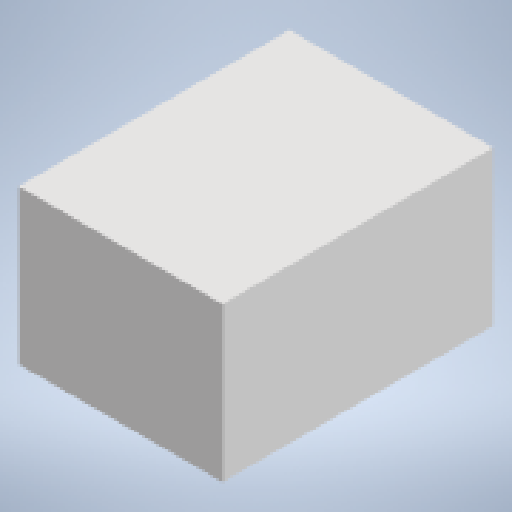
# Autodesk Inventor part: деталь будет крепить ремень
Saved by Autodesk Inventor 2024.2 (Build 282272000, 272)
## iProperties
Created: 2026-02-03
Part Number: деталь будет крепить ремень
Material: Типовые
Document SubType Name: Modeling
Designer: katya_notebook
Density: 1 g/cm^3
Appearance: По умолчанию
Author: katya_notebook
Autodesk Inventor part; units mm, degrees
ref_plane "YZ Plane" through (0, 0, 0) normal (1, 0, 0) x (0, 1, 0)
ref_plane "XZ Plane" through (0, 0, 0) normal (0, 1, 0) x (-1, 0, 0)
ref_plane "XY Plane" through (0, 0, 0) normal (0, 0, 1) x (1, 0, 0)
sketch "Эскиз1" plane through (0, 0, 0) normal (0, 0, 1) x (1, 0, 0)
  line L0 (4.9701, 7.2976) -> (4.9701, 8.7976)
  line L1 (4.9701, 8.7976) -> (-3.0052, 8.7976)
  line L2 (-3.0052, 7.2976) -> (4.9701, 7.2976)
  line L3 (-3.0052, 8.7976) -> (-3.0052, 7.2976)
  line L4 (-3.0052, 5.7776) -> (4.9701, 5.7776)
  line L5 (4.9701, 5.7776) -> (4.9701, 4.2776)
  line L6 (4.9701, 4.2776) -> (-3.0052, 4.2776)
  line L7 (-3.0052, 4.2776) -> (-3.0052, 5.7776)
  line L8 (4.9701, 5.0276) -> (-5.8657, 5.0276)
  arc A0 (-3.0052, 2.7576) -> (-2.4573, 3.2802) centre (-3.0114, 3.3126) ccw
  line L9 (-3.0052, 2.7576) -> (-3.0104, 4.0302)
  line L10 (-3.0104, 4.0302) -> (-3.0104, 4.2776)
  line L11 (-1.0104, 4.2776) -> (-1.0104, 3.8676)
  arc A1 (-1.0104, 3.8676) -> (-1.0114, 3.8676) centre (-1.0114, 3.3126) ccw
  line L12 (-1.0114, 3.8676) -> (-1.0114, 2.7576)
  arc A2 (-1.5664, 3.311) -> (-1.0114, 2.7576) centre (-1.0114, 3.3126) ccw
  line L13 (-1.5664, 3.311) -> (-1.5664, 3.3135)
  arc A3 (-1.5647, 3.3559) -> (-1.5664, 3.3135) centre (-1.0114, 3.3126) ccw
  arc A4 (-1.5647, 3.3559) -> (-1.7142, 3.5176) centre (-1.7142, 3.3676) ccw
  line L14 (-1.7142, 3.5176) -> (-2.3054, 3.5176)
  arc A5 (-2.3054, 3.5176) -> (-2.4554, 3.3676) centre (-2.3054, 3.3676) ccw
  line L15 (-2.4554, 3.3676) -> (-2.4554, 3.2802)
  line L16 (-2.4554, 3.2802) -> (-2.4573, 3.2802)
  arc A6 (-1.0114, 2.7576) -> (-0.4635, 3.2802) centre (-1.0175, 3.3126) ccw
  line L17 (-1.0114, 2.7576) -> (-1.0166, 4.0302)
  line L18 (-1.0166, 4.0302) -> (-1.0166, 4.2776)
  line L19 (0.9834, 4.2776) -> (0.9834, 3.8676)
  arc A7 (0.9834, 3.8676) -> (0.9825, 3.8676) centre (0.9825, 3.3126) ccw
  line L20 (0.9825, 3.8676) -> (0.9825, 2.7576)
  arc A8 (0.4275, 3.311) -> (0.9825, 2.7576) centre (0.9825, 3.3126) ccw
  line L21 (0.4275, 3.311) -> (0.4275, 3.3135)
  arc A9 (0.4291, 3.3559) -> (0.4275, 3.3135) centre (0.9825, 3.3126) ccw
  arc A10 (0.4291, 3.3559) -> (0.2796, 3.5176) centre (0.2796, 3.3676) ccw
  line L22 (0.2796, 3.5176) -> (-0.3116, 3.5176)
  arc A11 (-0.3116, 3.5176) -> (-0.4616, 3.3676) centre (-0.3116, 3.3676) ccw
  line L23 (-0.4616, 3.3676) -> (-0.4616, 3.2802)
  line L24 (-0.4616, 3.2802) -> (-0.4635, 3.2802)
  arc A12 (0.9825, 2.7576) -> (1.5304, 3.2802) centre (0.9763, 3.3126) ccw
  line L25 (0.9825, 2.7576) -> (0.9772, 4.0302)
  line L26 (0.9772, 4.0302) -> (0.9772, 4.2776)
  line L27 (2.9772, 4.2776) -> (2.9772, 3.8676)
  arc A13 (2.9772, 3.8676) -> (2.9763, 3.8676) centre (2.9763, 3.3126) ccw
  line L28 (2.9763, 3.8676) -> (2.9763, 2.7576)
  arc A14 (2.4213, 3.311) -> (2.9763, 2.7576) centre (2.9763, 3.3126) ccw
  line L29 (2.4213, 3.311) -> (2.4213, 3.3135)
  arc A15 (2.423, 3.3559) -> (2.4213, 3.3135) centre (2.9763, 3.3126) ccw
  arc A16 (2.423, 3.3559) -> (2.2734, 3.5176) centre (2.2734, 3.3676) ccw
  line L30 (2.2734, 3.5176) -> (1.6822, 3.5176)
  arc A17 (1.6822, 3.5176) -> (1.5322, 3.3676) centre (1.6822, 3.3676) ccw
  line L31 (1.5322, 3.3676) -> (1.5322, 3.2802)
  line L32 (1.5322, 3.2802) -> (1.5304, 3.2802)
  arc A18 (2.9763, 2.7576) -> (3.5242, 3.2802) centre (2.9701, 3.3126) ccw
  line L33 (2.9763, 2.7576) -> (2.9711, 4.0302)
  line L34 (2.9711, 4.0302) -> (2.9711, 4.2776)
  line L35 (4.9711, 4.2776) -> (4.9711, 3.8676)
  arc A19 (4.9711, 3.8676) -> (4.9701, 3.8676) centre (4.9701, 3.3126) ccw
  line L36 (4.9701, 3.8676) -> (4.9701, 2.7576)
  arc A20 (4.4151, 3.311) -> (4.9701, 2.7576) centre (4.9701, 3.3126) ccw
  line L37 (4.4151, 3.311) -> (4.4151, 3.3135)
  arc A21 (4.4168, 3.3559) -> (4.4151, 3.3135) centre (4.9701, 3.3126) ccw
  arc A22 (4.4168, 3.3559) -> (4.2673, 3.5176) centre (4.2673, 3.3676) ccw
  line L38 (4.2673, 3.5176) -> (3.6761, 3.5176)
  arc A23 (3.6761, 3.5176) -> (3.5261, 3.3676) centre (3.6761, 3.3676) ccw
  line L39 (3.5261, 3.3676) -> (3.5261, 3.2802)
  line L40 (3.5261, 3.2802) -> (3.5242, 3.2802)
  line L41 (4.9701, 2.7576) -> (-3.0052, 2.7576)
  line L42 (-3.0052, 2.7576) -> (-3.0052, 1.2576)
  line L43 (-3.0052, 1.2576) -> (4.9701, 1.2576)
  line L44 (4.9701, 1.2576) -> (4.9701, 2.7576)
  line L45 (-2.3054, 3.5176) -> (5.394, 3.5176)
  line L46 (4.9701, 3.7226) -> (4.3774, 3.7226)
  arc A24 (-0.4635, 3.755) -> (-1.0114, 4.2776) centre (-1.0175, 3.7226) ccw
  line L47 (0.9825, 4.2776) -> (0.9772, 3.005)
  line L48 (0.9825, 3.1676) -> (0.9825, 4.2776)
  line L49 (-1.0114, 4.2776) -> (-1.0166, 3.005)
  arc A25 (-2.4573, 3.755) -> (-3.0052, 4.2776) centre (-3.0114, 3.7226) ccw
  line L50 (-1.0114, 3.1676) -> (-1.0114, 4.2776)
  arc A26 (-1.5664, 3.7217) -> (-1.5647, 3.6793) centre (-1.0114, 3.7226) ccw
  line L51 (-1.5664, 3.7241) -> (-1.5664, 3.7217)
  arc A27 (-1.0114, 4.2776) -> (-1.5664, 3.7241) centre (-1.0114, 3.7226) ccw
  arc A28 (-1.7142, 3.5176) -> (-1.5647, 3.6793) centre (-1.7142, 3.6676) ccw
  arc A29 (1.5304, 3.755) -> (0.9825, 4.2776) centre (0.9763, 3.7226) ccw
  arc A30 (2.4213, 3.7217) -> (2.423, 3.6793) centre (2.9763, 3.7226) ccw
  arc A31 (2.9763, 4.2776) -> (2.4213, 3.7241) centre (2.9763, 3.7226) ccw
  line L52 (2.9763, 4.2776) -> (2.9711, 3.005)
  arc A32 (-2.4554, 3.6676) -> (-2.3054, 3.5176) centre (-2.3054, 3.6676) ccw
  line L53 (-2.4554, 3.6676) -> (-2.4554, 3.755)
  line L54 (-2.4554, 3.755) -> (-2.4573, 3.755)
  arc A33 (0.9825, 4.2776) -> (0.4275, 3.7241) centre (0.9825, 3.7226) ccw
  line L55 (0.4275, 3.7241) -> (0.4275, 3.7217)
  arc A34 (0.4275, 3.7217) -> (0.4291, 3.6793) centre (0.9825, 3.7226) ccw
  arc A35 (-0.4616, 3.6676) -> (-0.3116, 3.5176) centre (-0.3116, 3.6676) ccw
  line L56 (-0.4616, 3.755) -> (-0.4635, 3.755)
  arc A36 (0.2796, 3.5176) -> (0.4291, 3.6793) centre (0.2796, 3.6676) ccw
  line L57 (2.9763, 3.1676) -> (2.9763, 4.2776)
  line L58 (3.5261, 3.755) -> (3.5242, 3.755)
  line L59 (3.5261, 3.6676) -> (3.5261, 3.755)
  arc A37 (3.5261, 3.6676) -> (3.6761, 3.5176) centre (3.6761, 3.6676) ccw
  arc A38 (3.5242, 3.755) -> (2.9763, 4.2776) centre (2.9701, 3.7226) ccw
  arc A39 (4.9701, 4.2776) -> (4.4151, 3.7241) centre (4.9701, 3.7226) ccw
  line L60 (-0.4616, 3.6676) -> (-0.4616, 3.755)
  arc A40 (2.2734, 3.5176) -> (2.423, 3.6793) centre (2.2734, 3.6676) ccw
  line L61 (2.4213, 3.7241) -> (2.4213, 3.7217)
  line L62 (4.4151, 3.7241) -> (4.4151, 3.7217)
  arc A41 (4.4151, 3.7217) -> (4.4168, 3.6793) centre (4.9701, 3.7226) ccw
  arc A42 (1.5322, 3.6676) -> (1.6822, 3.5176) centre (1.6822, 3.6676) ccw
  line L63 (1.5322, 3.755) -> (1.5304, 3.755)
  arc A43 (4.2673, 3.5176) -> (4.4168, 3.6793) centre (4.2673, 3.6676) ccw
  line L64 (1.5322, 3.6676) -> (1.5322, 3.755)
  line L65 (4.9701, 3.3126) -> (4.3774, 3.3126)
  line L66 (4.9701, 4.2776) -> (4.9701, 5.7776)
  line L67 (4.9701, 5.7776) -> (-3.0052, 5.7776)
  line L68 (-3.0052, 5.7776) -> (-3.0052, 4.2776)
  arc A44 (-1.0114, 6.1876) -> (-1.0104, 6.1876) centre (-1.0114, 6.7426) ccw
  arc A45 (-0.4635, 6.775) -> (-1.0114, 7.2976) centre (-1.0175, 6.7426) ccw
  line L69 (0.9825, 7.2976) -> (0.9772, 6.025)
  line L70 (0.9825, 6.1876) -> (0.9825, 7.2976)
  line L71 (0.9772, 6.025) -> (0.9772, 5.7776)
  line L72 (-1.0104, 5.7776) -> (-1.0104, 6.1876)
  line L73 (-1.0114, 7.2976) -> (-1.0166, 6.025)
  line L74 (-1.0166, 6.025) -> (-1.0166, 5.7776)
  line L75 (-3.0104, 6.025) -> (-3.0104, 5.7776)
  line L76 (-3.0052, 7.2976) -> (-3.0104, 6.025)
  arc A46 (-2.4573, 6.775) -> (-3.0052, 7.2976) centre (-3.0114, 6.7426) ccw
  line L77 (-1.0114, 6.1876) -> (-1.0114, 7.2976)
  arc A47 (-1.5664, 6.7417) -> (-1.5647, 6.6993) centre (-1.0114, 6.7426) ccw
  line L78 (-1.5664, 6.7441) -> (-1.5664, 6.7417)
  arc A48 (-1.0114, 7.2976) -> (-1.5664, 6.7441) centre (-1.0114, 6.7426) ccw
  arc A49 (-1.7142, 6.5376) -> (-1.5647, 6.6993) centre (-1.7142, 6.6876) ccw
  line L79 (0.9834, 5.7776) -> (0.9834, 6.1876)
  arc A50 (0.9825, 6.1876) -> (0.9834, 6.1876) centre (0.9825, 6.7426) ccw
  arc A51 (1.5304, 6.775) -> (0.9825, 7.2976) centre (0.9763, 6.7426) ccw
  arc A52 (2.4213, 6.7417) -> (2.423, 6.6993) centre (2.9763, 6.7426) ccw
  arc A53 (2.9763, 7.2976) -> (2.4213, 6.7441) centre (2.9763, 6.7426) ccw
  line L80 (2.9763, 7.2976) -> (2.9711, 6.025)
  line L81 (2.9772, 5.7776) -> (2.9772, 6.1876)
  line L82 (2.9711, 6.025) -> (2.9711, 5.7776)
  line L83 (-1.7142, 6.5376) -> (-2.3054, 6.5376)
  arc A54 (-2.4554, 6.6876) -> (-2.3054, 6.5376) centre (-2.3054, 6.6876) ccw
  line L84 (-2.4554, 6.6876) -> (-2.4554, 6.775)
  line L85 (-2.4554, 6.775) -> (-2.4573, 6.775)
  arc A55 (0.9825, 7.2976) -> (0.4275, 6.7441) centre (0.9825, 6.7426) ccw
  line L86 (0.4275, 6.7441) -> (0.4275, 6.7417)
  arc A56 (0.4275, 6.7417) -> (0.4291, 6.6993) centre (0.9825, 6.7426) ccw
  line L87 (0.2796, 6.5376) -> (-0.3116, 6.5376)
  arc A57 (-0.4616, 6.6876) -> (-0.3116, 6.5376) centre (-0.3116, 6.6876) ccw
  line L88 (-0.4616, 6.775) -> (-0.4635, 6.775)
  arc A58 (0.2796, 6.5376) -> (0.4291, 6.6993) centre (0.2796, 6.6876) ccw
  line L89 (2.9763, 6.1876) -> (2.9763, 7.2976)
  line L90 (3.5261, 6.775) -> (3.5242, 6.775)
  line L91 (3.5261, 6.6876) -> (3.5261, 6.775)
  arc A59 (3.5261, 6.6876) -> (3.6761, 6.5376) centre (3.6761, 6.6876) ccw
  arc A60 (3.5242, 6.775) -> (2.9763, 7.2976) centre (2.9701, 6.7426) ccw
  line L92 (4.2673, 6.5376) -> (3.6761, 6.5376)
  arc A61 (4.9701, 7.2976) -> (4.4151, 6.7441) centre (4.9701, 6.7426) ccw
  line L93 (4.9711, 5.7776) -> (4.9711, 6.1876)
  line L94 (-0.4616, 6.6876) -> (-0.4616, 6.775)
  arc A62 (2.9763, 6.1876) -> (2.9772, 6.1876) centre (2.9763, 6.7426) ccw
  arc A63 (2.2734, 6.5376) -> (2.423, 6.6993) centre (2.2734, 6.6876) ccw
  line L95 (2.4213, 6.7441) -> (2.4213, 6.7417)
  line L96 (4.4151, 6.7441) -> (4.4151, 6.7417)
  arc A64 (4.4151, 6.7417) -> (4.4168, 6.6993) centre (4.9701, 6.7426) ccw
  line L97 (2.2734, 6.5376) -> (1.6822, 6.5376)
  arc A65 (1.5322, 6.6876) -> (1.6822, 6.5376) centre (1.6822, 6.6876) ccw
  line L98 (1.5322, 6.775) -> (1.5304, 6.775)
  arc A66 (4.2673, 6.5376) -> (4.4168, 6.6993) centre (4.2673, 6.6876) ccw
  arc A67 (4.9701, 6.1876) -> (4.9711, 6.1876) centre (4.9701, 6.7426) ccw
  line L99 (4.9701, 6.1876) -> (4.9701, 7.2976)
  line L100 (1.5322, 6.6876) -> (1.5322, 6.775)
  line L101 (4.9701, 7.2976) -> (-3.0052, 7.2976)
  line L102 (-3.0052, 7.2976) -> (-3.0052, 8.7976)
  line L103 (4.9701, 8.7976) -> (4.9701, 7.2976)
  line L104 (-2.3054, 6.5376) -> (5.394, 6.5376)
  line L105 (4.9701, 6.3326) -> (4.3774, 6.3326)
  line L106 (-1.5664, 6.331) -> (-1.5664, 6.3335)
  line L107 (-0.4616, 6.3002) -> (-0.4635, 6.3002)
  arc A68 (-0.3116, 6.5376) -> (-0.4616, 6.3876) centre (-0.3116, 6.3876) ccw
  arc A69 (-1.5647, 6.3759) -> (-1.5664, 6.3335) centre (-1.0114, 6.3326) ccw
  line L108 (-0.4616, 6.3876) -> (-0.4616, 6.3002)
  arc A70 (-1.0114, 5.7776) -> (-0.4635, 6.3002) centre (-1.0175, 6.3326) ccw
  arc A71 (-1.5664, 6.331) -> (-1.0114, 5.7776) centre (-1.0114, 6.3326) ccw
  arc A72 (-1.5647, 6.3759) -> (-1.7142, 6.5376) centre (-1.7142, 6.3876) ccw
  arc A73 (-2.3054, 6.5376) -> (-2.4554, 6.3876) centre (-2.3054, 6.3876) ccw
  line L109 (-2.4554, 6.3876) -> (-2.4554, 6.3002)
  line L110 (-2.4554, 6.3002) -> (-2.4573, 6.3002)
  arc A74 (-3.0052, 5.7776) -> (-2.4573, 6.3002) centre (-3.0114, 6.3326) ccw
  line L111 (0.9825, 5.7776) -> (0.9772, 7.0502)
  line L112 (0.9825, 6.8876) -> (0.9825, 5.7776)
  arc A75 (0.4291, 6.3759) -> (0.2796, 6.5376) centre (0.2796, 6.3876) ccw
  arc A76 (0.4291, 6.3759) -> (0.4275, 6.3335) centre (0.9825, 6.3326) ccw
  line L113 (0.4275, 6.331) -> (0.4275, 6.3335)
  arc A77 (0.4275, 6.331) -> (0.9825, 5.7776) centre (0.9825, 6.3326) ccw
  arc A78 (0.9825, 5.7776) -> (1.5304, 6.3002) centre (0.9763, 6.3326) ccw
  arc A79 (2.4213, 6.331) -> (2.9763, 5.7776) centre (2.9763, 6.3326) ccw
  arc A80 (2.423, 6.3759) -> (2.4213, 6.3335) centre (2.9763, 6.3326) ccw
  line L114 (1.5322, 6.3002) -> (1.5304, 6.3002)
  line L115 (1.5322, 6.3876) -> (1.5322, 6.3002)
  arc A81 (1.6822, 6.5376) -> (1.5322, 6.3876) centre (1.6822, 6.3876) ccw
  line L116 (2.4213, 6.331) -> (2.4213, 6.3335)
  arc A82 (2.423, 6.3759) -> (2.2734, 6.5376) centre (2.2734, 6.3876) ccw
  line L117 (2.9763, 5.7776) -> (2.9711, 7.0502)
  line L118 (2.9763, 6.8876) -> (2.9763, 5.7776)
  arc A83 (2.9763, 5.7776) -> (3.5242, 6.3002) centre (2.9701, 6.3326) ccw
  line L119 (3.5261, 6.3002) -> (3.5242, 6.3002)
  line L120 (3.5261, 6.3876) -> (3.5261, 6.3002)
  arc A84 (3.6761, 6.5376) -> (3.5261, 6.3876) centre (3.6761, 6.3876) ccw
  line L121 (-1.0114, 5.7776) -> (-1.0166, 7.0502)
  line L122 (-1.0114, 6.8876) -> (-1.0114, 5.7776)
  arc A85 (4.4151, 6.331) -> (4.9701, 5.7776) centre (4.9701, 6.3326) ccw
  line L123 (4.4151, 6.331) -> (4.4151, 6.3335)
  arc A86 (4.4168, 6.3759) -> (4.4151, 6.3335) centre (4.9701, 6.3326) ccw
  arc A87 (4.4168, 6.3759) -> (4.2673, 6.5376) centre (4.2673, 6.3876) ccw
  line L124 (4.9701, 6.7426) -> (4.3774, 6.7426)
  point P0 (0, 0)
  point P1 (-3.0052, 8.0476)
  point P2 (-3.0052, 5.0276)
  point P3 (4.9701, 8.0476)
  point P4 (0.4512, 3.5359)
  point P5 (-1.5427, 3.5359)
  point P6 (-3.5365, 3.5359)
  point P7 (-3.0052, 2.7576)
  point P8 (2.445, 3.5359)
  point P9 (-1.7142, 6.5376)
  point P10 (-1.0166, 5.7776)
  point P11 (-1.0104, 5.7776)
  point P12 (0.9772, 5.7776)
  point P13 (0.9834, 5.7776)
  point P14 (2.9711, 5.7776)
  point P15 (2.4213, 6.3335)
  point P16 (2.9772, 5.7776)
  point P17 (4.2673, 6.5376)
  point P18 (3.6761, 6.5376)
  point P19 (2.9772, 4.2776)
  point P20 (-3.0052, 4.2776)
  point P21 (-1.0166, 4.2776)
  point P22 (2.4213, 3.7217)
  point P23 (2.9711, 4.2776)
  point P24 (0.9834, 4.2776)
  point P25 (0.4275, 3.7217)
  point P26 (0.9772, 4.2776)
  point P27 (-1.0104, 4.2776)
  dimension "d0" = 1.5
  dimension "d10" = 0.41
  constraints: 250 end point, 228 symmetric about line, 176 point on circle, 88 centre point, 6 horizontal, 5 midpoint, 4 equal length, 4 parallel, 3 perpendicular, 2 point on line, 2 vertical, 2 vertical alignment, 64 other
  measures "d0" distance between parallel lines of L1 L2
  measures "d10" distance from line of L65.start L46
extrude "Выдавливание1" add sketch "Эскиз1" along normal blind 4.75 contours L2 L3 L1 L0 | A87 A86 A85 L4 A83 L120 A84 L92 | L5 L8 L7 L4 | L5 L6 L7 L8 | L97 A82 A80 L116 A79 L4 A78 L115 A81 | A39 A41 A43 L38 A37 L59 A38 L6 | L83 A72 A69 L106 A71 L4 A74 L109 A73 | L87 A75 A76 L113 A77 L4 A70 L108 A68 | L6 A27 L51 A26 A28 L14 A32 L53 A25 | A31 L61 A30 A40 L30 A42 L64 A29 L6 | L44 L43 L42 L41 | L6 A33 L55 A34 A36 L22 A35 L60 A24
sketch "Эскиз2" plane through (4.9701, 4.2776, 0) normal (1, 0, 0) x (0, 0, -1)
  line L0 (0, -1.52) -> (0, -3.02) projected
  line L1 (-4.75, 3.02) -> (-4.75, 4.52) projected
  line L2 (0, -3.02) -> (-4.75, -3.02)
  line L3 (-4.75, -3.02) -> (-4.75, 4.52)
  line L4 (-4.75, 4.52) -> (0, 4.52)
  line L5 (0, 4.52) -> (0, -3.02)
  point P0 (0, -4.2776)
  point P1 (0, -1.52)
  constraints: 8 end point, 2 parallel, 1 horizontal, 1 perpendicular
extrude "Выдавливание2" add sketch "Эскиз2" along normal blind 2
sketch "Эскиз3" plane through (0, 0, 4.75) normal (0, 0, 1) x (1, 0, 0)
  line L0 (-3.0052, 1.2576) -> (6.9701, 1.2576) projected
  line L1 (-3.0052, 8.7976) -> (6.9701, 8.7976) projected
  line L2 (6.9701, 1.2576) -> (-3.0052, 1.2576)
  line L3 (-3.0052, 1.2576) -> (-3.0052, 8.7976)
  line L4 (-3.0052, 8.7976) -> (6.9701, 8.7976)
  line L5 (6.9701, 8.7976) -> (6.9701, 1.2576)
  point P0 (0, 0)
  point P1 (-3.0052, 1.2576)
  point P2 (6.9701, 8.7976)
  constraints: 8 end point, 2 parallel, 1 horizontal, 1 perpendicular
extrude "Выдавливание3" add sketch "Эскиз3" along normal blind 2
ref_plane "РабПлоскость1" through (1.9948, 5.0311, -3.25) normal (0, 0, -1) x (-1, 0, 0)
